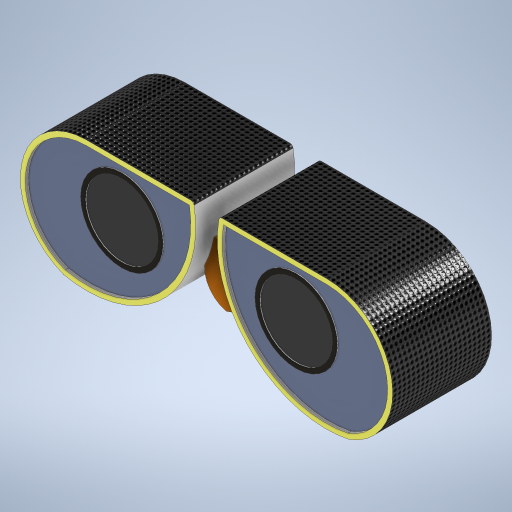
# Autodesk Inventor part: Project eyes
Saved by Autodesk Inventor 2024 (Build 280153000, 153)
## iProperties
Created: 2023-06-27
Part Number: Project eyes
Material: Generic
Document SubType Name: Modeling
Designer: hardi
Density: 1 g/cm^3
Appearance: Default
Author: hardi
Autodesk Inventor part; units mm, degrees
ref_plane "YZ Plane" through (0, 0, 0) normal (1, 0, 0) x (0, 1, 0)
ref_plane "XZ Plane" through (0, 0, 0) normal (0, 1, 0) x (-1, 0, 0)
ref_plane "XY Plane" through (0, 0, 0) normal (0, 0, 1) x (1, 0, 0)
sketch "Sketch1" plane through (0, 0, 0) normal (0, 0, 1) x (1, 0, 0)
  line L0 (1.6571, 0) -> (65, 0)
  arc A0 (78.6808, -77.5877) -> (65, 0) centre (65, -40) ccw
  line L1 (65, -40) -> (78.6808, -77.5877) construction
  line L2 (65, -40) -> (65, 0) construction
  arc A1 (-0.3126, -1.6535) -> (78.6808, -77.5877) centre (64.6893, -13.0878) ccw
  arc A2 (1.6571, 0) -> (-0.3126, -1.6535) centre (1.6571, -2) ccw
  line L3 (65, -3) -> (2.5022, -3)
  arc A3 (2.5022, -3) -> (77.8443, -74.699) centre (64.6893, -13.0878) ccw
  arc A4 (77.8443, -74.699) -> (65, -3) centre (65, -40) ccw
  point P0 (0, 0)
  dimension "d4" = 65
  dimension "d5" = 160
  dimension "d6" = 66
  dimension "d8" = 2
  dimension "d11" = 3
  constraints: 11 point on circle, 8 end point, 5 centre point, 2 tangent, 1 horizontal, 1 point on line, 2 other
  measures "d4" distance of point (0, 0) L0.end
  measures "d5" angle of L1 L2
  measures "d6" radius of A1
  measures "d8" radius of A2
  measures "d11" distance between parallel lines of L0 L3
extrude "Extrusion1" add sketch "Sketch1" against normal blind 60 contours L0 A0 A1 A2 | A4 A3 L3
extrude "Extrusion2" cut sketch "Sketch1" against normal blind 2 contours A4 A3 L3
sketch "Sketch3" plane through (0, 0, -2) normal (0, 0, 1) x (1, 0, 0)
  circle A0 centre (45, -33) radius 25
  circle A1 centre (45, -33) radius 22
  point P0 (0, 0)
  dimension "d14" = 50
  dimension "d15" = 3
  constraints: 2 centre point
  measures "d14" diameter of A0
  measures "d15" radial gap between concentric circles of A0 A1
extrude "Extrusion3" add sketch "Sketch3" along normal blind 0.5
ref_plane "Work Plane1" through (0, 0, -32) normal (0, 0, 1) x (1, 0, 0)
sketch "Sketch4" plane through (0, 0, -32) normal (0, 0, 1) x (1, 0, 0)
  arc A0 (-0.3126, -1.6535) -> (78.6808, -77.5877) centre (64.6893, -13.0878) ccw projected
  line L0 (-0.3126, -24.5221) -> (-7.8126, -24.5221)
  line L1 (-7.8126, -24.5221) -> (-7.8126, -59.5221)
  arc A1 (-7.8126, -59.5221) -> (5.3698, -42.0221) centre (-11.6048, -42.9504) ccw
  point P0 (0, 0)
  dimension "d19" = 7.5
  dimension "d20" = 35
  dimension "d21" = 17
  constraints: 4 end point, 4 point on circle, 1 centre point, 1 horizontal, 1 perpendicular
  measures "d19" distance of L0.start L0.end
  measures "d20" distance of L0.end L1.end
  measures "d21" radius of A1
extrude "Extrusion4" add sketch "Sketch4" along normal mid plane 40
mirror "Mirror1" about plane through (-7.8126, -24.5221, -32) normal (-1, 0, 0)
body "Solid1"
